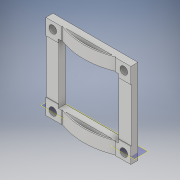
# Autodesk Inventor part: 30_Sampleclamp_generic
Saved by Autodesk Inventor 2019 (Build 230136000, 136)
## iProperties
Created: 2019-09-11
Part Number: 30_Sampleclamp_generic
Material: Generic
Document SubType Name: Modeling
Designer: marsikovabarbora
Density: 1 g/cm^3
Appearance: Default
Author: marsikovabarbora
Autodesk Inventor part; units mm, degrees
ref_plane "YZ Plane" through (0, 0, 0) normal (1, 0, 0) x (0, 1, 0)
ref_plane "XZ Plane" through (0, 0, 0) normal (0, 1, 0) x (-1, 0, 0)
ref_plane "XY Plane" through (0, 0, 0) normal (0, 0, 1) x (1, 0, 0)
sketch "Sketch1" plane through (0, 0, 0) normal (0, 0, 1) x (1, 0, 0)
  line L0 (-16.9, -16.9) -> (-16.9, 16.9)
  line L1 (-16.9, 16.9) -> (16.9, 16.9)
  line L2 (16.9, 16.9) -> (16.9, -16.9)
  line L3 (16.9, -16.9) -> (-16.9, -16.9)
  circle A0 centre (-20, 20) radius 2.75
  circle A1 centre (20, -20) radius 2.75
  circle A2 centre (20, 20) radius 2.75
  circle A3 centre (-20, -20) radius 2.75
  line L4 (-22.9, 22.9) -> (22.9, 22.9)
  line L5 (-22.9, -22.9) -> (-22.9, 22.9)
  line L6 (22.9, -22.9) -> (-22.9, -22.9)
  line L7 (22.9, 22.9) -> (22.9, -22.9)
  line L8 (23.9, 23.9) -> (-23.9, 23.9)
  line L9 (-23.9, 23.9) -> (-23.9, -23.9)
  line L10 (-23.9, -23.9) -> (23.9, -23.9)
  line L11 (23.9, -23.9) -> (23.9, 23.9)
  point P0 (0, 0)
  point P1 (0, 0)
  dimension "d8" = 1
  constraints: 24 end point, 4 centre point, 3 other
  measures "d8" distance between parallel lines of L4 L8
extrude "Extrusion1" add sketch "Sketch1" along normal blind 4 contours A0 | A1 | A2 | A3 | L4 L7 L6 L5 | L11 L10 L9 L8
sketch "Sketch2" plane through (0, 0, 4) normal (0, 0, 1) x (1, 0, 0)
  line L0 (-16.9, 16.9) -> (16.9, 16.9) projected
  line L1 (16.9, 16.9) -> (16.9, -16.9) projected
  line L2 (16.9, -16.9) -> (-16.9, -16.9) projected
  line L3 (-16.9, -16.9) -> (-16.9, 16.9) projected
  line L4 (-16.9, -16.9) -> (-16.9, 16.9)
  line L5 (-16.9, 16.9) -> (16.9, 16.9)
  line L6 (16.9, 16.9) -> (16.9, -16.9)
  line L7 (16.9, -16.9) -> (-16.9, -16.9)
  circle A0 centre (-20, 20) radius 2.15
  circle A1 centre (20, -20) radius 2.15
  circle A2 centre (20, 20) radius 2.15
  circle A3 centre (-20, -20) radius 2.15
  line L8 (-22.9, 22.9) -> (22.9, 22.9)
  line L9 (-22.9, -22.9) -> (-22.9, 22.9)
  line L10 (22.9, -22.9) -> (-22.9, -22.9)
  line L11 (22.9, 22.9) -> (22.9, -22.9)
  point P0 (0, 0)
  point P1 (0, 0)
  dimension "d2" = 4.3
  dimension "d3" = 4.3
  dimension "d4" = 4.3
  dimension "d5" = 4.3
  constraints: 16 end point, 4 centre point, 4 other
  measures "d2" diameter of A0
  measures "d3" diameter of A2
  measures "d4" diameter of A3
  measures "d5" diameter of A1
extrude "Extrusion2" cut sketch "Sketch2" against normal through all contours A0 | A1 | A2 | A3
ref_plane "Work Plane1" through (-20, -20, 4) normal (0, -1, 0) x (1, 0, 0)
sketch "Sketch3" plane through (-20, -20, 4) normal (0, -1, 0) x (1, 0, 0)
  line L0 (2.15, -4) -> (-2.15, -4) projected
  line L1 (-2.15, 0) -> (2.15, 0) projected
  line L2 (43.9, -4) -> (-3.9, -4) projected
  line L3 (-3.9, -4) -> (-3.9, 0) projected
  line L4 (43.9, 0) -> (-3.9, 0) projected
  line L5 (43.9, -4) -> (43.9, 0) projected
  line L6 (0, 2.9614) -> (0, -7.6552) construction
  arc A0 (-2.15, 0) -> (0, -4.1992) centre (0, -1.5492) ccw
  line L7 (0, 1.1008) -> (0, -4.1992)
  arc A1 (0, 1.1008) -> (-2.15, 0) centre (0, -1.5492) ccw
  arc A2 (0, -4.1992) -> (0, 1.1008) centre (0, -1.5492) ccw
  point P0 (20, -4)
  point P1 (0, -4)
  dimension "d10" = 5.3
  constraints: 8 point on circle, 5 end point, 4 point on line, 3 centre point, 1 midpoint, 1 vertical
  measures "d10" diameter of A0
revolve "Revolution1" cut sketch "Sketch3" angle 360 about axis through (-20, -20, 5.1008) along (0, 0, -1) contours A2 L7 L0 | L0 L7 L1 A2 | L1 L7 A2
pattern_linear "Rectangular Pattern1" count 2 spacing 40 along (1, 0, 0) count 2 spacing 40 along (0, 1, 0) of "Revolution1"
sketch "Sketch4" plane through (0, 0, 4) normal (0, 0, 1) x (1, 0, 0)
  circle A0 centre (20, 20) radius 2.15 projected
  circle A1 centre (-20, 20) radius 2.15 projected
  circle A2 centre (20, -20) radius 2.15 projected
  circle A3 centre (-20, -20) radius 2.15 projected
  line L0 (-16.9, 16.9) -> (16.9, 16.9) projected
  line L1 (16.9, 16.9) -> (16.9, -16.9) projected
  line L2 (16.9, -16.9) -> (-16.9, -16.9) projected
  line L3 (-16.9, -16.9) -> (-16.9, 16.9) projected
  line L4 (23.9, 23.9) -> (-23.9, 23.9) projected
  line L5 (-23.9, 23.9) -> (-23.9, -23.9) projected
  line L6 (-23.9, -23.9) -> (23.9, -23.9) projected
  line L7 (23.9, -23.9) -> (23.9, 23.9) projected
  line L8 (-33.46, 0) -> (33.46, 0) construction
  line L9 (0, -33.46) -> (0, 33.46) construction
  line L10 (-15, 23.9) -> (15, 23.9)
  line L11 (15, 23.9) -> (15, 16.9)
  line L12 (15, 16.9) -> (-15, 16.9)
  line L13 (-15, 16.9) -> (-15, 23.9)
  line L14 (-23.9, -15) -> (-23.9, 15)
  line L15 (-16.9, -15) -> (-23.9, -15)
  line L16 (-16.9, 15) -> (-16.9, -15)
  line L17 (-23.9, 15) -> (-16.9, 15)
  line L18 (15, -23.9) -> (-15, -23.9)
  line L19 (15, -16.9) -> (15, -23.9)
  line L20 (-15, -16.9) -> (15, -16.9)
  line L21 (-15, -23.9) -> (-15, -16.9)
  line L22 (23.9, 15) -> (23.9, -15)
  line L23 (16.9, 15) -> (23.9, 15)
  line L24 (16.9, -15) -> (16.9, 15)
  line L25 (23.9, -15) -> (16.9, -15)
  point P0 (0, 0)
  dimension "d18" = 30
  dimension "d21" = 360
  constraints: 32 end point, 2 parallel, 2 point on line, 1 horizontal, 1 perpendicular, 34 other
  measures "d18" distance between parallel lines of L11 L13
extrude "Extrusion3" cut sketch "Sketch4" against normal blind 0.3 contours L13 L4 L11 L0 | L3 L15 L5 L17 | L23 L7 L25 L1 | L2 L19 L6 L21
sketch "Sketch5" plane through (-23.9, 23.9, 0) normal (0, 1, 0) x (1, 0, 0)
  line L0 (38.9, -3.7) -> (38.9, -4) construction
  line L1 (47.8, -4) -> (38.9, -4) construction
  line L2 (47.8, 0) -> (47.8, -4) construction
  line L3 (47.8, 0) -> (0, 0) construction
  line L4 (0, 0) -> (0, -4) construction
  line L5 (8.9, -4) -> (0, -4) construction
  line L6 (8.9, -4) -> (8.9, -3.7) construction
  line L7 (8.9, -3.7) -> (38.9, -3.7) construction
  line L8 (23.9, 0) -> (23.9, -19.2449) construction
  line L9 (38.9, -3.7) -> (8.9, -3.7) projected
  line L10 (8.9, -3.7) -> (23.9, -9.5) construction
  line L11 (23.9, -9.5) -> (38.9, -3.7) construction
  spline S0 degree 2 poles (8.9, -3.7) (23.9, -9.5) (38.9, -3.7) knots 1 1 1 2 2 2
  line L12 (23.9, -3.7) -> (23.9, -6.6) construction
  line L13 (9.225, -3.0751) -> (8.9, -3.7)
  line L14 (38.9, -4) -> (38.9, -3.7) projected
  line L15 (38.575, -3.0751) -> (38.9, -3.7)
  spline S1 degree 5 poles (9.225, -3.0751) (12.0305, -4.1545) (14.9217, -5.0099) (17.888, -5.6036) (23.9, -6.1963) (29.912, -5.6036) (32.8783, -5.0099) (35.7695, -4.1545) (38.575, -3.0751) knots 0 0 0 0 0 0 0.5 0.5 0.5 1 1 1 1 1 1
  dimension "d26" = 0.7
  dimension "d25" = 2.9
  constraints: 8 end point, 2 point on line, 1 horizontal alignment, 1 midpoint, 1 vertical, 6 other
  measures "d25" distance from line of L12.end L7
extrude "Extrusion4" add sketch "Sketch5" against normal up to surface (7 mm away) contours S0 L9 S1 | L9 S1 L15 | L13 S1 L9
sketch "Sketch6" plane through (-23.9, -23.9, 0) normal (0, -1, 0) x (1, 0, 0)
  line L0 (36.8497, 3.7) -> (10.9503, 3.7) projected
  spline S0 degree 5 poles (10.9504, 3.7) (13.4491, 4.5486) (16.01, 5.2141) (18.6221, 5.6716) (23.9, 6.1284) (29.1779, 5.6716) (31.79, 5.2141) (34.3509, 4.5486) (36.8496, 3.7) knots 0 0 0 0 0 0 0.5 0.5 0.5 1 1 1 1 1 1 projected
  spline S1 degree 2 poles (38.9, 3.7) (23.9, 9.5) (8.9, 3.7) knots 0 0 0 1 1 1 projected
  line L1 (8.9, 3.7) -> (8.9, 4) projected
  line L2 (7, 4) -> (8.9, 4) projected
  line L3 (7, 0) -> (7, 4) projected
  line L4 (40.8, 0) -> (7, 0) projected
  line L5 (40.8, 0) -> (40.8, 4) projected
  line L6 (38.9, 4) -> (40.8, 4) projected
  line L7 (38.9, 4) -> (38.9, 3.7) projected
  point P0 (23.9, 0)
  constraints: 2 horizontal alignment
extrude "Extrusion5" add sketch "Sketch6" against normal up to surface (7 mm away)
equation "\"d3\" = d2"
equation "\"d4\" = d2"
equation "\"d5\" = d2"
body "Solid1"
